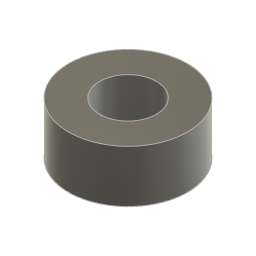
Pul (Autodesk Fusion 360 design; units mm, degrees)
Autodesk Fusion 360 part; units mm, degrees
sketch "Eskiz1" plane through (0, 0, 0) normal (0, 1, 0) x (1, 0, 0)
  circle A0 centre (6.2737, -4.9582) radius 1.2
  circle A1 centre (6.2737, -4.9582) radius 2.5
  dimension "d1" = 2.4
  dimension "d2" = 5
  constraint concentric A0 A1
  measures "d1" diameter of A0
  measures "d2" diameter of A1
extrude "Ekstrüde Et1" add sketch "Eskiz1" along normal blind 2.2
equation "d1 = 2 mm + 0.4 mm"
